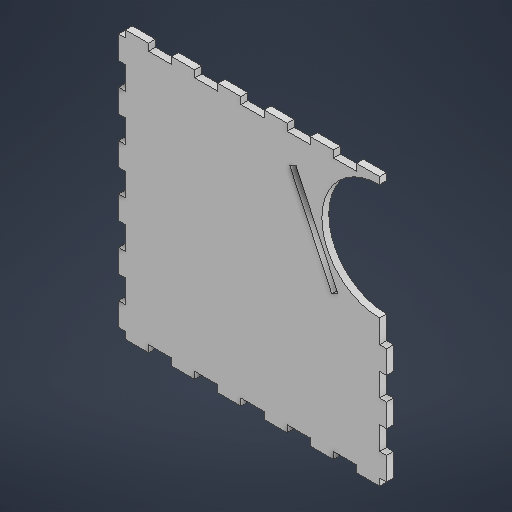
# Autodesk Inventor part: ParedPantalla
Saved by Autodesk Inventor 2026 (Build 300175000, 175)
## iProperties
Created: 2026-04-21
Part Number: ParedPantalla
Material: Generic
Document SubType Name: Modeling
Designer: juana
Density: 1 g/cm^3
Appearance: Default
Author: juana
Autodesk Inventor part; units mm, degrees
ref_plane "YZ Plane" through (0, 0, 0) normal (1, 0, 0) x (0, 1, 0)
ref_plane "XZ Plane" through (0, 0, 0) normal (0, 1, 0) x (-1, 0, 0)
ref_plane "XY Plane" through (0, 0, 0) normal (0, 0, 1) x (1, 0, 0)
sketch "Sketch1" plane through (0, 0, 0) normal (0, 0, 1) x (1, 0, 0)
  line L0 (0, 110) -> (110, 110)
  line L1 (110, 60) -> (110, 0)
  line L2 (110, 0) -> (0, 0)
  line L3 (0, 0) -> (0, 110)
  arc A0 (110, 110) -> (110, 60) centre (110, 85) ccw
  line L4 (73.8274, 98.9712) -> (73.8274, 60) construction
  line L5 (73.8274, 60) -> (92, 60) construction
  line L6 (73.8274, 98.9712) -> (92, 60)
  line L7 (92, 60) -> (73.8274, 98.9712) construction
  line L8 (73.8274, 98.9712) -> (71.1085, 97.7034)
  line L9 (71.1085, 97.7034) -> (89.2811, 58.7321)
  line L10 (89.2811, 58.7321) -> (92, 60)
  line L11 (0, 0) -> (10, 0)
  line L12 (10, 0) -> (10, -3)
  line L13 (10, -3) -> (0, -3)
  line L14 (0, -3) -> (0, 0)
  line L15 (30, 0) -> (30, -3)
  line L16 (20, 0) -> (30, 0)
  line L17 (20, -3) -> (20, 0)
  line L18 (30, -3) -> (20, -3)
  line L19 (50, 0) -> (50, -3)
  line L20 (40, 0) -> (50, 0)
  line L21 (40, -3) -> (40, 0)
  line L22 (50, -3) -> (40, -3)
  line L23 (70, 0) -> (70, -3)
  line L24 (60, 0) -> (70, 0)
  line L25 (60, -3) -> (60, 0)
  line L26 (70, -3) -> (60, -3)
  line L27 (90, 0) -> (90, -3)
  line L28 (80, 0) -> (90, 0)
  line L29 (80, -3) -> (80, 0)
  line L30 (90, -3) -> (80, -3)
  line L31 (110, 0) -> (110, -3)
  line L32 (100, 0) -> (110, 0)
  line L33 (100, -3) -> (100, 0)
  line L34 (110, -3) -> (100, -3)
  line L35 (10, 113) -> (10, 110)
  line L36 (0, 113) -> (10, 113)
  line L37 (0, 110) -> (0, 113)
  line L38 (10, 110) -> (0, 110)
  line L39 (30, 113) -> (30, 110)
  line L40 (20, 113) -> (30, 113)
  line L41 (20, 110) -> (20, 113)
  line L42 (30, 110) -> (20, 110)
  line L43 (50, 113) -> (50, 110)
  line L44 (40, 113) -> (50, 113)
  line L45 (40, 110) -> (40, 113)
  line L46 (50, 110) -> (40, 110)
  line L47 (70, 113) -> (70, 110)
  line L48 (60, 113) -> (70, 113)
  line L49 (60, 110) -> (60, 113)
  line L50 (70, 110) -> (60, 110)
  line L51 (90, 113) -> (90, 110)
  line L52 (80, 113) -> (90, 113)
  line L53 (80, 110) -> (80, 113)
  line L54 (90, 110) -> (80, 110)
  line L55 (110, 113) -> (110, 110)
  line L56 (100, 113) -> (110, 113)
  line L57 (100, 110) -> (100, 113)
  line L58 (110, 110) -> (100, 110)
  point P0 (0, 0)
  dimension "d1" = 110
  dimension "d2" = 110
  dimension "d3" = 110
  dimension "d4" = 25
  dimension "d6" = 18.1726
  dimension "d7" = 38.9712
  dimension "d8" = 18
  dimension "d9" = 3
  dimension "d12" = 3
  dimension "d13" = 10
  dimension "d16" = 20
  dimension "d19" = 113
  constraints: 118 end point, 6 perpendicular, 4 parallel, 3 horizontal, 2 point on circle, 2 vertical, 2 vertical alignment, 1 centre point, 1 coincident, 1 collinear, 1 horizontal alignment, 88 other
  measures "d1" distance of L2.end L0.start
  measures "d2" distance of L1.end L2.end
  measures "d3" distance of L0.start L0.end
  measures "d4" radius of A0
  measures "d6" distance of L4.end L5.end
  measures "d7" distance of L4.start L4.end
  measures "d8" distance from line of L1 L5.end
  measures "d9" distance of L4.start L8.end
  measures "d12" distance of L13.end L2.end
  measures "d13" distance of L12.end L13.end
  measures "d16" distance of L11.end L15.start
  measures "d19" distance of L11.end L35.start
extrude "Extrusion1" add sketch "Sketch1" along normal blind 3
sketch "Sketch2" plane through (0, 0, 3) normal (0, 0, 1) x (1, 0, 0)
  line L0 (0, 0) -> (-3, 0)
  line L1 (-3, 0) -> (-3, 10)
  line L2 (-3, 10) -> (0, 10)
  line L3 (0, 10) -> (0, 0)
  line L4 (0, 113) -> (0, -3) construction
  line L5 (90, 0) -> (100, 0) construction
  line L6 (0, 20) -> (-3, 20)
  line L7 (-3, 20) -> (-3, 30)
  line L8 (-3, 30) -> (0, 30)
  line L9 (0, 30) -> (0, 20)
  line L10 (0, 40) -> (-3, 40)
  line L11 (-3, 40) -> (-3, 50)
  line L12 (-3, 50) -> (0, 50)
  line L13 (0, 50) -> (0, 40)
  line L14 (0, 60) -> (-3, 60)
  line L15 (-3, 60) -> (-3, 70)
  line L16 (-3, 70) -> (0, 70)
  line L17 (0, 70) -> (0, 60)
  line L18 (0, 80) -> (-3, 80)
  line L19 (-3, 80) -> (-3, 90)
  line L20 (-3, 90) -> (0, 90)
  line L21 (0, 90) -> (0, 80)
  line L22 (0, 100) -> (-3, 100)
  line L23 (-3, 100) -> (-3, 110)
  line L24 (-3, 110) -> (0, 110)
  line L25 (0, 110) -> (0, 100)
  line L26 (113, 10) -> (113, 0)
  line L27 (113, 0) -> (110, 0)
  line L28 (110, 0) -> (110, 10)
  line L29 (110, 10) -> (113, 10)
  line L30 (0, 30) -> (0, 20)
  line L31 (0, 20) -> (-3, 20)
  line L32 (-3, 20) -> (-3, 30)
  line L33 (-3, 30) -> (0, 30)
  line L34 (113, 30) -> (113, 20)
  line L35 (113, 20) -> (110, 20)
  line L36 (110, 20) -> (110, 30)
  line L37 (110, 30) -> (113, 30)
  line L38 (0, 50) -> (0, 40)
  line L39 (0, 40) -> (-3, 40)
  line L40 (-3, 40) -> (-3, 50)
  line L41 (-3, 50) -> (0, 50)
  line L42 (113, 50) -> (113, 40)
  line L43 (113, 40) -> (110, 40)
  line L44 (110, 40) -> (110, 50)
  line L45 (110, 50) -> (113, 50)
  dimension "d22" = 3
  dimension "d23" = 10
  dimension "d26" = 20
  dimension "d33" = 113
  dimension "d36" = 20
  constraints: 88 end point, 2 horizontal, 2 parallel, 2 vertical, 1 perpendicular, 80 other
  measures "d22" distance of L0.start L0.end
  measures "d23" distance of L0.end L1.end
  measures "d26" distance of L1.end L7.end
  measures "d33" distance of L0.start L26.end
  measures "d36" distance of L0.start L30.end
extrude "Extrusion2" add sketch "Sketch2" against normal blind 3
body "Solid1"
